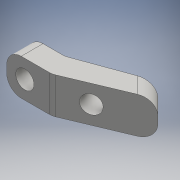
# Autodesk Inventor part: rpi_mount
Saved by Autodesk Inventor 2016 (Build 200138000, 138)
## iProperties
Created: 2016-09-22
Part Number: rpi_mount
Material: Generic
Document SubType Name: Modeling
Designer: Jakub
Density: 1 g/cm^3
Appearance: Default
Author: Jakub
Autodesk Inventor part; units mm, degrees
ref_plane "YZ Plane" through (0, 0, 0) normal (1, 0, 0) x (0, 1, 0)
ref_plane "XZ Plane" through (0, 0, 0) normal (0, 1, 0) x (-1, 0, 0)
ref_plane "XY Plane" through (0, 0, 0) normal (0, 0, 1) x (1, 0, 0)
sketch "Sketch1" plane through (0, 0, 0) normal (0, 0, 1) x (1, 0, 0)
  line L0 (-2.5, -1.5) -> (2.5, -1.5)
  line L1 (2.5, -1.5) -> (2.5, 1.5)
  line L2 (2.5, 1.5) -> (-2.5, 1.5)
  line L3 (-2.5, 1.5) -> (-2.5, -1.5)
  line L4 (-2.5, -1.5) -> (2.5, 1.5) construction
  line L5 (2.5, -1.5) -> (-2.5, 1.5) construction
  line L6 (2.5, 1.5) -> (11.8969, 4.9202)
  line L7 (2.5, 1.5) -> (12.5, 1.5) construction
  line L8 (11.8969, 4.9202) -> (14.0182, 2.7989)
  line L9 (14.0182, 2.7989) -> (3.7426, -1.5)
  line L10 (3.7426, -1.5) -> (2.5, -1.5)
  point P0 (0, 0)
  dimension "d0" = 5
  dimension "d1" = 3
  dimension "d2" = 10
  dimension "d3" = 20
  dimension "d4" = 3
  constraints: 22 end point, 3 horizontal, 2 midpoint, 2 parallel, 1 equal length, 1 perpendicular
  measures "d0" distance of L2.end L1.end
  measures "d1" distance of L1.end L0.end
  measures "d2" distance of L1.end L6.end
  measures "d3" angle of L7 L6
  measures "d4" distance of L6.end L8.end
extrude "Extrusion1" add sketch "Sketch1" along normal blind 5
sketch "Sketch2" plane through (-2.5, 1.5, 0) normal (0, 1, 0) x (1, 0, 0)
  line L0 (2.5, 0) -> (2.5, -5)
  line L1 (0, -5) -> (6.2426, -5) projected
  circle A0 centre (2.5, -2.5) radius 1.25
  dimension "d7" = 2.5
  constraints: 2 end point, 1 centre point, 1 midpoint, 1 point on line, 1 vertical
  measures "d7" diameter of A0
extrude "Extrusion2" cut sketch "Sketch2" against normal blind 5
fillet "Fillet1" radius 2 2 edges at (2.5, 1.5, 2.5) (3.7426, -1.5, 2.5)
sketch "Sketch3" plane through (11.8969, 4.9202, 0) normal (-0.342, 0.9397, 0) x (-0.9397, -0.342, 0)
  line L0 (-1.2679, 0) -> (-1.2679, 5) projected
  line L1 (-1.2679, 2.5) -> (5.7321, 2.5)
  circle A0 centre (5.7321, 2.5) radius 1.25
  point P0 (12.8623, 0)
  dimension "d11" = 7
  dimension "d12" = 2.5
  constraints: 2 end point, 1 centre point, 1 coincident, 1 horizontal, 1 midpoint
  measures "d11" distance of L1.start L1.end
  measures "d12" diameter of A0
extrude "Extrusion3" cut sketch "Sketch3" against normal up to next
fillet "Fillet2" radius 2 4 edges at (12.9576, 3.8595, 5) (12.9576, 3.8595, 0) (-2.5, 0, 5) (-2.5, 0, 0)
body "Solid1"
